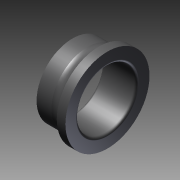
# Autodesk Inventor part: 7205 BEP_PART1
Saved by Autodesk Inventor 2011 SP1 (Build 150282100, 282)
## iProperties
Created: 2016-06-15
Part Number: 7205 BEP_PART1
Catalog Web Link: www.cadenas.de
Description: -Angular contact ball bearings, single row
Vendor: SKF
Document SubType Name: Modeling
Designer: psAdmin
Manufacturer: SKF
Mass: 5.06572 g
Surface Area: 35.6364 cm^2
Volume: 5.06572 cm^3
Density: 1 g/cm^3
Category: PARTsolutions
Company: SKF
Title: 7205 BEP_PART1
Author: Cadenas PARTsolutions
Comments: Angular contact ball bearings, single row
PSOL_IDENT_0: {$CADENAS_DATA\23d-libs\skf\bearings_units_and_housings\ball_bearings\angular_contact_ball_bearings\
PSOL_IDENT_1: ba1_001_101.prj},198 {VTYP=3D},{NB=7205 BEP_PART1},{LINA=7205 BEP_PART1},{NN=BA1_001_101_PART1},{NOP
PSOL_IDENT_2: RJ=TRUE},{DATE=14.06.2016 09:57:36},{GEOMDATE=25.04.2016 09:30:22},{VERSION=},{LINEID=141940},{LINES
PSOL_IDENT_3: UBID=-1},{WBVAR=}  {NB=7205 BEP_PART1},{LINA=7205 BEP_PART1},{KT=DUMMY},{PRODUCTID=1210010205},{DESI
PSOL_IDENT_4: GNATION=7205 BEP},{DD=25.000},{D=52.000},{B=15.0000},{C1=-1000000015047466219876688855040.000},{DD1=
PSOL_IDENT_5: 36.100},{DD2A=30.870},{DD2=30.87},{D3=-1000000015047466219876688855040.000},{D1=41.570},{D2A=46.270}
PSOL_IDENT_6: ,{D2=46.27},{D4=-1000000015047466219876688855040.000},{D5=46.800},{R12=1.000},{R34=0.600},{AA=24.000
PSOL_IDENT_7: },{LOAD1=14.800},{LOAD2=9.300},{LOAD3=0.400},{SPEED1=15000},{SPEED2=15000},{MASS=0.130},{PITCH=38.50
PSOL_IDENT_8: 0},{DW=7.938},{Z=13.000},{II=1.000},{ALPHA=40.000},{TYPEID=121001},{R5R=0.6},{R34L=1},{IRH=1},{ORH=1
PSOL_IDENT_9: },{D4H=1},{TAXONOMY=1},{DESIGN=acbb1},{MAPPING=BCZ50,DESIGNATION|IRD01,DD|ORD10,D|BCW30,B|ORL02,C1|I
PSOL_IDENT_10: RD30,DD1|IRD31,DD2A|ORD30,D1|ORD31,D2A|ORD15,D3|ORD43,D4|ORD44,D5|IRL03,R12|ORL05,R34|BCL30,AA|BCC02
PSOL_IDENT_11: ,LOAD1|BCC16,LOAD2|BCC12,LOAD3|BCC43,SPEED1|BCC45,SPEED2|BCM01,MASS|BCD50,PITCH|RBD10,DW|BCN81,Z|BCN
PSOL_IDENT_12: 80,II|BCA50,ALPHA},{DESIGNLIST=acbb1,acbb1f,design_ba1_001_101_1},{SORT=DD},{PIM=7205 BEP}
NT: Angular contact ball bearings, single row
NB: 7205 BEP_PART1
NBSYN: $DESIGNATION._PART1
LINA: 7205 BEP_PART1
DESIGNATION: 7205 BEP
DD: 25.000
D: 52.000
B: 15.0000
DD2A: 30.870
D2A: 46.270
LOAD1: 14.800
LOAD2: 9.300
LOAD3: 0.400
SPEED1: 15000
SPEED2: 15000
SUPPLIER: SKF
ARTICLENO: 7205 BEP_PART1
BOMINFO: 7205 BEP_PART1
CREATOR: CADENAS GmbH
Autodesk Inventor part; units mm, degrees
ref_plane "YZ Plane" through (0, 0, 0) normal (1, 0, 0) x (0, 1, 0)
ref_plane "XZ Plane" through (0, 0, 0) normal (0, 1, 0) x (-1, 0, 0)
ref_plane "XY Plane" through (0, 0, 0) normal (0, 0, 1) x (1, 0, 0)
sketch "Sketch_1" plane through (0, 0, 0) normal (0, 0, 1) x (1, 0, 0)
  line L0 (15, 0) -> (0, 0)
  line L1 (0, 15.435) -> (0, 13.5)
  arc A0 (0, 13.5) -> (1, 12.5) centre (1, 13.5) ccw
  line L2 (1, 12.5) -> (14, 12.5)
  arc A1 (14, 12.5) -> (15, 13.5) centre (14, 13.5) ccw
  line L3 (15, 13.5) -> (15, 18.05)
  line L4 (15, 18.05) -> (11.2832, 18.05)
  arc A2 (6.4051, 15.435) -> (11.2832, 18.05) centre (7.5, 19.25) ccw
  line L5 (6.4051, 15.435) -> (0, 15.435)
  constraints: 12 end point, 6 point on circle, 3 centre point
revolve "Revolution1" add sketch "Sketch_1" angle 360 about axis through (15, 0, 0) along (1, 0, 0)
body "Solid1"
